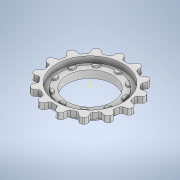
# Autodesk Inventor part: Bánh răng dẫn xích
Saved by Autodesk Inventor 2022 (Build 260153000, 153)
## iProperties
Created: 2022-04-22
Part Number: Bánh răng dẫn xích
Material: Generic
Document SubType Name: Modeling
Designer: duyne
Density: 1 g/cm^3
Appearance: Default
Author: duyne
Autodesk Inventor part; units mm, degrees
ref_plane "YZ Plane" through (0, 0, 0) normal (1, 0, 0) x (0, 1, 0)
ref_plane "XZ Plane" through (0, 0, 0) normal (0, 1, 0) x (-1, 0, 0)
ref_plane "XY Plane" through (0, 0, 0) normal (0, 0, 1) x (1, 0, 0)
sketch "Sketch2" plane through (0, 0, 0) normal (0, 1, 0) x (-1, 0, 0)
  circle A0 centre (0, 0) radius 19.5
  dimension "d8" = 39
  constraints: 1 centre point, 1 coincident
  measures "d8" diameter of A0
extrude "Extrusion2" add sketch "Sketch2" along normal mid plane 2.73
sketch "Sketch3" plane through (0, 1.365, 0) normal (0, 1, 0) x (1, 0, 0)
  line L0 (0, 16.5) -> (1, 16.5)
  arc A0 (1, 16.5) -> (1.8734, 17.013) centre (1, 17.5) ccw
  line L1 (1.8734, 17.013) -> (3.3956, 19.743)
  line L2 (4.269, 20.256) -> (6.0629, 20.256)
  arc A1 (4.269, 20.256) -> (3.3956, 19.743) centre (4.269, 19.256) ccw
  line L3 (-5.4666, 20.256) -> (-6.0629, 20.256)
  line L4 (0, 0) -> (0, 22.2293)
  line L5 (0, 16.5) -> (-1, 16.5)
  arc A2 (-1.8734, 17.013) -> (-1, 16.5) centre (-1, 17.5) ccw
  line L6 (-1.8734, 17.013) -> (-3.3956, 19.743)
  line L7 (-4.269, 20.256) -> (-6.0629, 20.256)
  arc A3 (-3.3956, 19.743) -> (-4.269, 20.256) centre (-4.269, 19.256) ccw
  line L8 (-6.0629, 20.256) -> (6.0629, 20.256)
  dimension "d11" = 1
  dimension "d12" = 1
  dimension "d16" = 2.73
  dimension "d24" = 1
  constraints: 18 end point, 8 point on circle, 6 symmetric about line, 4 centre point, 4 tangent, 3 horizontal, 1 vertical, 1 vertical alignment, 2 other
  measures "d11" radius of A0
  measures "d12" radius of A1
  measures "d16" vertical distance of L1.start L1.end
  measures "d24" distance of L0.start L0.end
extrude "Extrusion3" cut sketch "Sketch3" against normal through all
pattern_circular "Circular Pattern1" count 14 over 360 about axis through (0, 0, 0) along (0, 1, 0) of "Extrusion3"
fillet "Fillet1" radius 1.3 1 edges at (3.12, 0, -19.2488)
fillet "Fillet2" radius 1.3 1 edges at (-5.5407, 0, -18.6963)
fillet "Fillet3" radius 1.3 1 edges at (-13.104, 0, -14.4407)
fillet "Fillet4" radius 1.3 1 edges at (-18.0719, 0, -7.325)
fillet "Fillet5" radius 1.3 1 edges at (-19.4604, 0, 1.2415)
fillet "Fillet6" radius 1.3 1 edges at (-16.9946, 0, 9.5621)
fillet "Fillet7" radius 1.3 1 edges at (-11.1628, 0, 15.9888)
fillet "Fillet8" radius 1.3 1 edges at (-3.12, 0, 19.2488)
fillet "Fillet9" radius 1.3 1 edges at (5.5407, 0, 18.6963)
fillet "Fillet10" radius 1.3 4 edges at (13.104, 0, 14.4407) (18.0719, 0, 7.325) (19.4604, 0, -1.2415) (16.9946, 0, -9.5621)
fillet "Fillet11" radius 1.3 1 edges at (11.1628, 0, -15.9888)
fillet "Fillet12" radius 1.3 1 edges at (-3.12, 0, -19.2488)
fillet "Fillet13" radius 1.3 13 edges at (13.104, 0, -14.4407) (18.0719, 0, -7.325) (19.4604, 0, 1.2415) (16.9946, 0, 9.5621) (11.1628, 0, 15.9888) (3.12, 0, 19.2488) (-5.5407, 0, 18.6963) (-13.104, 0, 14.4407) (-18.0719, 0, 7.325) (-19.4604, 0, -1.2415) (-16.9946, 0, -9.5621) (-11.1628, 0, -15.9888) (5.5407, 0, -18.6963)
sketch "Sketch5" plane through (0, 0, 0) normal (0, 1, 0) x (-1, 0, 0)
  point P0 (0, 0)
sketch "Sketch7" plane through (0, 1.365, 0) normal (0, 1, 0) x (1, 0, 0)
  point P0 (0, 0)
sketch "Sketch8" plane through (0, 1.365, 0) normal (0, 1, 0) x (1, 0, 0)
  circle A0 centre (0, 0) radius 15.25
  dimension "d49" = 30.5
  constraints: 1 centre point, 1 coincident
  measures "d49" diameter of A0
extrude "Extrusion4" cut sketch "Sketch8" against normal through all
sketch "Sketch9" plane through (0, -1.365, 0) normal (0, -1, 0) x (1, 0, 0)
  circle A0 centre (0, 0) radius 15.25 projected
  circle A1 centre (0, 0) radius 15.95
  dimension "d52" = 31.9
  constraints: 1 centre point, 1 coincident
  measures "d52" diameter of A1
extrude "Extrusion5" add sketch "Sketch9" along normal blind 2.86 contours A0
chamfer "Chamfer1" distance 2 angle 45 1 edges at (-15.25, -4.225, 0)
sketch "Sketch12" plane through (0, -1.365, 0) normal (0, 1, 0) x (1, 0, 0)
  circle A0 centre (0, 0) radius 13.25
  dimension "d65" = 26.5
  constraints: 1 centre point, 1 coincident
  measures "d65" diameter of A0
extrude "Extrusion8" add sketch "Sketch12" along normal blind 0.53
sketch "Sketch13" plane through (0, -0.835, 0) normal (0, 1, 0) x (1, 0, 0)
  circle A0 centre (0, 0) radius 10.5
  dimension "d68" = 21
  constraints: 1 centre point, 1 coincident
  measures "d68" diameter of A0
extrude "Extrusion9" cut sketch "Sketch13" against normal blind 32.725
sketch "Sketch14" plane through (0, -0.835, 0) normal (0, 1, 0) x (1, 0, 0)
  circle A0 centre (0, 0) radius 13.25 projected
  line L0 (-1.62, -13.1506) -> (1.62, -13.1506)
  arc A1 (1.62, -13.1506) -> (-1.62, -13.1506) centre (0, -13.1597) ccw
  circle A2 centre (0, 0) radius 13.25 projected
  circle A3 centre (0, 0) radius 15.25 projected
  point P0 (0, -12.02)
  constraints: 4 point on circle, 2 end point, 1 centre point
extrude "Extrusion10" add sketch "Sketch14" along normal blind 0.75 contours A1 L0
fillet "Fillet14" radius 0.25 1 edges at (0, -0.085, 11.5397)
pattern_circular "Circular Pattern2" count 10 over 360 about axis through (0, -1.365, 0) along (0, 1, 0) of "Extrusion10"
fillet "Fillet15" radius 0.25 5 edges at (1.5468, -0.1582, 13.1506) (1.62, -0.585, 13.1506) (-1.5468, -0.1582, 13.1506) (-1.62, -0.585, 13.1506) (0, -0.085, 13.1506)
fillet "Fillet16" radius 0.25 2 edges at (-6.7829, -0.085, 9.3358) (-7.7297, -0.085, 10.6391)
fillet "Fillet17" radius 0.25 2 edges at (-12.507, -0.085, 4.0638) (-10.9749, -0.085, 3.566)
fillet "Fillet18" radius 0.25 2 edges at (-10.9749, -0.085, -3.566) (-12.507, -0.085, -4.0638)
fillet "Fillet19" radius 0.25 2 edges at (-7.7297, -0.085, -10.6391) (-6.7829, -0.085, -9.3358)
fillet "Fillet20" radius 0.25 2 edges at (0, -0.085, -13.1506) (0, -0.085, -11.5397)
fillet "Fillet21" radius 0.25 2 edges at (7.7297, -0.085, -10.6391) (6.7829, -0.085, -9.3358)
fillet "Fillet22" radius 0.25 2 edges at (12.507, -0.085, -4.0638) (10.9749, -0.085, -3.566)
fillet "Fillet23" radius 0.25 2 edges at (12.507, -0.085, 4.0638) (10.9749, -0.085, 3.566)
fillet "Fillet24" radius 0.25 2 edges at (7.7297, -0.085, 10.6391) (6.7829, -0.085, 9.3358)
body "Solid2"
